screw_wheel_20_m4 (Autodesk Fusion 360 design; units mm, degrees)
Autodesk Fusion 360 part; units mm, degrees
note: some values were not read from the file. Set by a fixed rule: which sketch regions a step uses.
sketch "Sketch1" plane through (0, 0, 0) normal (0, 1, 0) x (1, 0, 0)
  circle A0 centre (0, 0) radius 10
  circle A1 centre (0, 0) radius 2.1
  dimension "d1" = 20
  dimension "d2" = 4.2
  constraint coincident A0.centre A1.centre
  constraint concentric A0 A1
  measures "d1" diameter of A0
  measures "d2" diameter of A1
extrude "Extrude1" add sketch "Sketch1" along normal blind 4
fillet "Fillet1" radius 1 2 edges at (-9.3233, 0, 3.6162) (-9.3233, 4, 3.6162)
sketch "Sketch2" plane through (0, 0, 0) normal (0, -1, 0) x (1, 0, 0)
  circle A0 centre (0, 0) radius 2.1
  circle A1 centre (0, 0) radius 9
  circle A2 centre (0, 0) radius 10
  circle A3 centre (0, 10) radius 0.75
  circle A4 centre (-1.1702, 9.3269) radius 0.6
  circle A5 centre (1.1702, 9.3269) radius 0.6
  dimension "d7" = 1.5
  dimension "d8" = 1.2
  constraint coincident A2 A3.centre
  constraint vertical A0.centre A3.centre
  constraint tangent A2 A4
  constraint tangent A3 A4
  constraint tangent A3 A5
  constraint tangent A2 A5
  constraint equal A4 A5
  measures "d7" diameter of A3
  measures "d8" diameter of A4
extrude "Extrude2" cut sketch "Sketch2" against normal through all contours A2 A3 A4 | A2 A3 | A2 A3 A5 picked at (0, 9.7479)
pattern_circular "C-Pattern1" count 23 over 360 about axis through (0, 1.75, 0) along (0, 1, 0) of "Extrude2"
sketch "Sketch3" plane through (0, 0, 0) normal (0, -1, 0) x (1, 0, 0)
  circle A0 centre (0, 0) radius 2.1
  circle A1 centre (0, 0) radius 9
  line L0 (-2.0785, 3.6) -> (-4.1569, 0)
  line L1 (-4.1569, 0) -> (-2.0785, -3.6)
  line L2 (-2.0785, -3.6) -> (2.0785, -3.6)
  line L3 (2.0785, -3.6) -> (4.1569, 0)
  line L4 (4.1569, 0) -> (2.0785, 3.6)
  line L5 (2.0785, 3.6) -> (-2.0785, 3.6)
  dimension "d12" = 7.2
  constraint coincident A0.centre A1.centre
  constraint horizontal L0.end A0.centre
  measures "d12" distance of L2 L5
extrude "Extrude3" cut sketch "Sketch3" against normal blind 3.5 contours L0 L1 L2 L3 L4 L5
